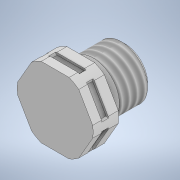
# Autodesk Inventor part: Vent Port M12
Saved by Autodesk Inventor 2021 (Build 250183000, 183)
## iProperties
Created: 2019-11-15
Part Number: Vent Port M12
Material: Generic
Document SubType Name: Modeling
Designer: jgray
Density: 1 g/cm^3
Appearance: Default
Vendor: Farnell
Stock Number: 2911974
Author: jgray
Autodesk Inventor part; units mm, degrees
ref_plane "YZ Plane" through (0, 0, 0) normal (1, 0, 0) x (0, 1, 0)
ref_plane "XZ Plane" through (0, 0, 0) normal (0, 1, 0) x (-1, 0, 0)
sketch "Sketch1" plane through (0, 0, 0) normal (0, 0, 1) x (1, 0, 0)
  line L0 (5.35023, 6.73313) -> (8.506177, 1.26687)
  line L1 (8.506177, -1.26687) -> (5.35023, -6.73313)
  line L2 (3.155947, -8) -> (-3.155947, -8)
  line L3 (-5.35023, -6.73313) -> (-8.506177, -1.26687)
  line L4 (-8.506177, 1.26687) -> (-5.35023, 6.73313)
  line L5 (-3.155947, 8) -> (3.155947, 8)
  arc A0 (5.35023, 6.73313) -> (3.155947, 8) centre (0, 0) ccw
  arc A1 (8.506177, -1.26687) -> (8.506177, 1.26687) centre (0, 0) ccw
  arc A2 (3.155947, -8) -> (5.35023, -6.73313) centre (0, 0) ccw
  arc A3 (-5.35023, -6.73313) -> (-3.155947, -8) centre (0, 0) ccw
  arc A4 (-3.155947, 8) -> (-5.35023, 6.73313) centre (0, 0) ccw
  arc A5 (-8.506177, 1.26687) -> (-8.506177, -1.26687) centre (0, 0) ccw
  dimension "d0" = 16
  constraints: 12 end point, 12 point on circle, 6 centre point, 2 coincident, 7 other
  measures "d0" distance between parallel lines of L2 L5
sketch "Sketch1 outline for Extrusion1" plane through (0, 0, 0) normal (0, 0, 1) x (1, 0, 0)
  arc A0 (8.506177, -1.26687) -> (8.506177, 1.26687) centre (0, 0) ccw
  line L0 (5.35023, -6.73313) -> (8.506177, -1.26687)
  arc A1 (3.155947, -8) -> (5.35023, -6.73313) centre (0, 0) ccw
  line L1 (-3.155947, -8) -> (3.155947, -8)
  arc A2 (-5.35023, -6.73313) -> (-3.155947, -8) centre (0, 0) ccw
  line L2 (-8.506177, -1.26687) -> (-5.35023, -6.73313)
  arc A3 (-8.506177, 1.26687) -> (-8.506177, -1.26687) centre (0, 0) ccw
  line L3 (-5.35023, 6.73313) -> (-8.506177, 1.26687)
  arc A4 (-3.155947, 8) -> (-5.35023, 6.73313) centre (0, 0) ccw
  line L4 (3.155947, 8) -> (-3.155947, 8)
  arc A5 (5.35023, 6.73313) -> (3.155947, 8) centre (0, 0) ccw
  line L5 (8.506177, 1.26687) -> (5.35023, 6.73313)
extrude "Extrusion1" add sketch "Sketch1 outline for Extrusion1" along normal blind 5.8
shell "Shell2" thickness 0.5 removed faces 0
ref_plane "Work Plane1" through (0, 0, 3.8) normal (0, 0, 1) x (1, 0, 0)
sketch "Sketch2" plane through (0, 0, 3.8) normal (0, 0, 1) x (1, 0, 0)
  line L0 (-4.965485, 6.399528) -> (-8.024896, 1.100472)
  arc A0 (-8.024896, 1.100472) -> (-8.024896, -1.100472) centre (0, 0) ccw
  line L1 (-8.024896, -1.100472) -> (-4.965485, -6.399528)
  arc A1 (-4.965485, -6.399528) -> (-3.059412, -7.5) centre (0, 0) ccw
  line L2 (-3.059412, -7.5) -> (3.059412, -7.5)
  arc A2 (3.059412, -7.5) -> (4.965485, -6.399528) centre (0, 0) ccw
  line L3 (4.965485, -6.399528) -> (8.024896, -1.100472)
  arc A3 (8.024896, -1.100472) -> (8.024896, 1.100472) centre (0, 0) ccw
  line L4 (8.024896, 1.100472) -> (4.965485, 6.399528)
  arc A4 (4.965485, 6.399528) -> (3.059412, 7.5) centre (0, 0) ccw
  line L5 (3.059412, 7.5) -> (-3.059412, 7.5)
  arc A5 (-3.059412, 7.5) -> (-4.965485, 6.399528) centre (0, 0) ccw
  arc A6 (-3.614518, 8) -> (3.614518, 8) centre (0, 11.454744) ccw
  line L6 (3.059412, 7.5) -> (-3.059412, 7.5)
  line L7 (-3.614518, 8) -> (3.614518, 8)
  line L8 (3.155947, 8) -> (-3.155947, 8)
  arc A7 (-8.735462, 0.869735) -> (-5.120944, 7.130265) centre (-9.920099, 5.727372) ccw
  line L9 (-8.735462, 0.869735) -> (-5.120944, 7.130265)
  arc A8 (-5.120944, -7.130265) -> (-8.735462, -0.869735) centre (-9.920099, -5.727372) ccw
  line L10 (-5.120944, -7.130265) -> (-8.735462, -0.869735)
  arc A9 (3.614518, -8) -> (-3.614518, -8) centre (0, -11.454744) ccw
  line L11 (3.614518, -8) -> (-3.614518, -8)
  arc A10 (8.735462, -0.869735) -> (5.120944, -7.130265) centre (9.920099, -5.727372) ccw
  line L12 (8.735462, -0.869735) -> (5.120944, -7.130265)
  arc A11 (5.120944, 7.130265) -> (8.735462, 0.869735) centre (9.920099, 5.727372) ccw
  line L13 (5.120944, 7.130265) -> (8.735462, 0.869735)
  point P0 (-8.024896, 1.100472)
  point P1 (-4.965485, 6.399528)
  point P2 (-5.35023, 6.73313)
  point P3 (-8.506177, 1.26687)
  point P4 (-4.965485, -6.399528)
  point P5 (-8.024896, -1.100472)
  point P6 (-8.506177, -1.26687)
  point P7 (-5.35023, -6.73313)
  point P8 (3.059412, -7.5)
  point P9 (-3.059412, -7.5)
  point P10 (-3.155947, -8)
  point P11 (3.155947, -8)
  point P12 (8.024896, -1.100472)
  point P13 (4.965485, -6.399528)
  point P14 (5.35023, -6.73313)
  point P15 (8.506177, -1.26687)
  point P16 (4.965485, 6.399528)
  point P17 (8.024896, 1.100472)
  point P18 (8.506177, 1.26687)
  point P19 (5.35023, 6.73313)
  point P20 (-8.024896, 1.100472)
  point P21 (8.024896, -1.100472)
  point P22 (4.965485, -6.399528)
  point P23 (8.024896, 1.100472)
  dimension "d7" = 10
  dimension "d10" = 360
  constraints: 24 point on circle, 12 end point, 6 centre point, 1 collinear, 55 other
  measures "d7" diameter of A6
sketch "Sketch2 outline for Extrusion2" plane through (0, 0, 3.8) normal (0, 0, 1) x (1, 0, 0)
  line L0 (-5.120944, 7.130265) -> (-8.735462, 0.869735)
  arc A0 (-4.965485, 6.399528) -> (-5.120944, 7.130265) centre (-9.920099, 5.727372) ccw
  line L1 (-8.024896, 1.100472) -> (-4.965485, 6.399528)
  arc A1 (-8.735462, 0.869735) -> (-8.024896, 1.100472) centre (-9.920099, 5.727372) ccw
  line L2 (-8.735462, -0.869735) -> (-5.120944, -7.130265)
  arc A2 (-5.120944, -7.130265) -> (-8.735462, -0.869735) centre (-9.920099, -5.727372) ccw
  line L3 (-3.614518, -8) -> (3.614518, -8)
  arc A3 (3.614518, -8) -> (-3.614518, -8) centre (0, -11.454744) ccw
  line L4 (5.120944, -7.130265) -> (8.735462, -0.869735)
  arc A4 (4.965485, -6.399528) -> (5.120944, -7.130265) centre (9.920099, -5.727372) ccw
  line L5 (8.024896, -1.100472) -> (4.965485, -6.399528)
  arc A5 (8.735462, -0.869735) -> (8.024896, -1.100472) centre (9.920099, -5.727372) ccw
  line L6 (8.735462, 0.869735) -> (5.120944, 7.130265)
  arc A6 (8.024896, 1.100472) -> (8.735462, 0.869735) centre (9.920099, 5.727372) ccw
  line L7 (4.965485, 6.399528) -> (8.024896, 1.100472)
  arc A7 (5.120944, 7.130265) -> (4.965485, 6.399528) centre (9.920099, 5.727372) ccw
  line L8 (3.614518, 8) -> (-3.614518, 8)
  arc A8 (3.059412, 7.5) -> (3.614518, 8) centre (0, 11.454744) ccw
  line L9 (-3.059412, 7.5) -> (3.059412, 7.5)
  arc A9 (-3.614518, 8) -> (-3.059412, 7.5) centre (0, 11.454744) ccw
extrude "Extrusion2" cut sketch "Sketch2 outline for Extrusion2" against normal blind 1.5
sketch "Sketch3" plane through (0, 0, 0) normal (0, 0, -1) x (-1, 0, 0)
  circle A0 centre (0, 0) radius 5
  dimension "d14" = 10
  constraints: 1 centre point, 1 coincident
  measures "d14" diameter of A0
sketch "Sketch3 outline for Extrusion3" plane through (0, 0, 0) normal (0, 0, -1) x (-1, 0, 0)
  circle A0 centre (0, 0) radius 5
extrude "Extrusion3" add sketch "Sketch3 outline for Extrusion3" along normal blind 2
sketch "Sketch4" plane through (0, 0, -2) normal (0, 0, -1) x (-1, 0, 0)
  circle A0 centre (0, 0) radius 5.95
  dimension "d17" = 11.9
  constraints: 1 centre point, 1 coincident
  measures "d17" diameter of A0
sketch "Sketch4 outline for Extrusion4" plane through (0, 0, -2) normal (0, 0, -1) x (-1, 0, 0)
  circle A0 centre (0, 0) radius 5.95
extrude "Extrusion4" add sketch "Sketch4 outline for Extrusion4" along normal blind 8
chamfer "Chamfer1" distance 0.8 angle 45 2 edges at (5.95, 0, -2) (5.95, 0, -10)
thread "Thread1" size "M12x1.75" class "6g" standard "ANSI Metric M Profile" length 11
sketch "Sketch5" plane through (0, 0, -10) normal (0, 0, -1) x (-1, 0, 0)
  circle A0 centre (0, 0) radius 3.5
  dimension "d25" = 7
  constraints: 1 centre point, 1 coincident
  measures "d25" diameter of A0
sketch "Sketch5 outline for Extrusion5" plane through (0, 0, -10) normal (0, 0, -1) x (-1, 0, 0)
  circle A0 centre (0, 0) radius 3.5
extrude "Extrusion5" cut sketch "Sketch5 outline for Extrusion5" against normal blind 10
body "Solid1"
